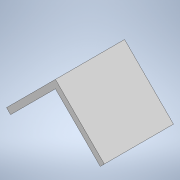
# Autodesk Inventor part: Tablero
Saved by Autodesk Inventor 2022 (Build 260153000, 153)
## iProperties
Created: 2022-08-25
Part Number: Tablero
Material: Generic
Document SubType Name: Modeling
Designer: Sebastian
Density: 1 g/cm^3
Appearance: Default
Author: Sebastian
Autodesk Inventor part; units mm, degrees
ref_plane "YZ Plane" through (0, 0, 0) normal (1, 0, 0) x (0, 1, 0)
ref_plane "XZ Plane" through (0, 0, 0) normal (0, 1, 0) x (-1, 0, 0)
ref_plane "XY Plane" through (0, 0, 0) normal (0, 0, 1) x (1, 0, 0)
sketch "Sketch1" plane through (0, 0, 0) normal (0, 0, 1) x (1, 0, 0)
  line L0 (0, 0) -> (-17.6777, 17.6777)
  line L1 (-17.6777, 17.6777) -> (194.4544, 229.8097)
  line L2 (-17.6777, 17.6777) -> (282.3223, 17.6777) construction
  line L3 (194.4544, 229.8097) -> (406.5864, 17.6777)
  line L4 (406.5864, 17.6777) -> (388.9087, 0)
  line L5 (388.9087, 0) -> (194.4544, 194.4544)
  line L6 (194.4544, 194.4544) -> (0, 0)
  dimension "d2" = 300
  dimension "d3" = 45
  dimension "d4" = 300
  dimension "d5" = 25
  constraints: 14 end point, 4 perpendicular, 1 equal length, 1 horizontal
  measures "d2" distance of L0.end L1.end
  measures "d3" angle of L2 L1
  measures "d4" distance of L1.end L3.end
  measures "d5" distance of L3.end L4.end
extrude "Extrusion1" add sketch "Sketch1" along normal blind 300
sketch "Sketch3" plane through (-17.6777, 17.6777, 0) normal (-0.7071, 0.7071, 0) x (-0.7071, -0.7071, 0)
  line L0 (-300, 0) -> (0, 0) projected
  line L1 (-180, 0) -> (-180, 300)
  line L2 (-300, 300) -> (0, 300) projected
  line L3 (-150, 0) -> (-180, 0)
  line L4 (-180, 0) -> (-180, 300)
  spline S0 degree 2 poles (-215.7606, 120.2254) (-207.5352, 120.2254) (-195.8732, 115.9437) (-188.4366, 107.8873) (-185, 96.3944) (-185, 88.4507) knots 0 0 0 1 2 3 4 4 4
  line L5 (-185, 88.4507) -> (-185, 74.1972)
  spline S1 degree 2 poles (-185, 74.1972) (-185, 72.6761) (-186.8028, 70.5915) (-188.831, 70.5915) knots 0 0 0 1 2 2 2
  line L6 (-188.831, 70.5915) -> (-240.8873, 70.5915)
  spline S2 degree 2 poles (-240.8873, 70.5915) (-242.9155, 70.5915) (-244.7183, 72.6761) (-244.7183, 74.1972) knots 0 0 0 1 2 2 2
  line L7 (-244.7183, 74.1972) -> (-244.7183, 89.5211)
  spline S3 degree 2 poles (-244.7183, 89.5211) (-244.7183, 97.5211) (-241, 108.6197) (-233.6197, 116.2817) (-222.8592, 120.2254) (-215.7606, 120.2254) knots 0 0 0 1 2 3 4 4 4
  spline S4 degree 2 poles (-215.3099, 107.662) (-219.5352, 107.662) (-226.8592, 105.6901) (-232.2113, 101.2958) (-235.1972, 94.4225) (-235.1972, 88.8451) knots 0 0 0 1 2 3 4 4 4
  line L8 (-235.1972, 88.8451) -> (-235.1972, 82.7042)
  line L9 (-235.1972, 82.7042) -> (-194.5775, 82.7042)
  line L10 (-194.5775, 82.7042) -> (-194.5775, 89.0141)
  spline S5 degree 2 poles (-194.5775, 89.0141) (-194.5775, 94.0282) (-197.169, 100.8451) (-202.3521, 105.4084) (-210.1268, 107.662) (-215.3099, 107.662) knots 0 0 0 1 2 3 4 4 4
  spline S6 degree 2 poles (-202.9155, 186.9296) (-198.1831, 186.9296) (-191.0845, 183.4366) (-186.3521, 177.4084) (-183.9296, 169.4084) (-183.9296, 164.8451) knots 0 0 0 1 2 3 4 4 4
  spline S7 degree 2 poles (-183.9296, 164.8451) (-183.9296, 161.7465) (-184.9437, 156.4507) (-186.4085, 152.3944) (-187.9859, 149.6338) (-189.169, 148.4507) (-191.4225, 147.9437) (-193.5634, 147.9437) knots 0 0 0 1 2 3 4 5 6 6 6
  spline S8 degree 2 poles (-193.5634, 147.9437) (-194.9718, 147.9437) (-196.9437, 148.1127) (-198.1268, 148.5634) (-198.6338, 149.2394) (-198.6338, 149.6901) knots 0 0 0 1 2 3 4 4 4
  spline S9 degree 2 poles (-198.6338, 149.6901) (-198.6338, 150.3662) (-197.1127, 152.6761) (-195.2535, 156.3944) (-193.7324, 161.5211) (-193.7324, 164.8451) knots 0 0 0 1 2 3 4 4 4
  spline S10 degree 2 poles (-193.7324, 164.8451) (-193.7324, 167.0986) (-194.8028, 170.5915) (-196.7183, 173.0141) (-199.5915, 174.3099) (-201.338, 174.3099) knots 0 0 0 1 2 3 4 4 4
  spline S11 degree 2 poles (-201.338, 174.3099) (-203.3662, 174.3099) (-206.2958, 172.1127) (-208.5493, 168.5634) (-210.5211, 164.0563) (-212.7183, 159.2113) (-215.5352, 154.7042) (-219.4789, 151.1549) (-224.831, 148.9577) (-228.5493, 148.9577) knots 0 0 0 1 2 3 4 5 6 7 8 8 8
  spline S12 degree 2 poles (-228.5493, 148.9577) (-232.8873, 148.9577) (-239.3662, 152.169) (-243.6479, 157.5211) (-245.7887, 164.9014) (-245.7887, 169.0141) knots 0 0 0 1 2 3 4 4 4
  spline S13 degree 2 poles (-245.7887, 169.0141) (-245.7887, 171.0986) (-245.169, 175.3803) (-244.0423, 179.0423) (-242.6338, 181.9155) (-241.7324, 182.8732) (-241.1127, 183.1549) (-240.0423, 183.3803) (-238.4085, 183.493) (-237.2254, 183.493) knots 0 0 0 1 2 3 4 5 6 7 8 8 8
  spline S14 degree 2 poles (-237.2254, 183.493) (-235.8732, 183.493) (-234.0141, 183.3803) (-232.831, 183.0423) (-232.2676, 182.4225) (-232.2676, 181.9155) knots 0 0 0 1 2 3 4 4 4
  spline S15 degree 2 poles (-232.2676, 181.9155) (-232.2676, 181.4084) (-233.5634, 179.2113) (-235.0845, 175.9437) (-236.3239, 171.7183) (-236.3239, 169.1831) knots 0 0 0 1 2 3 4 4 4
  spline S16 degree 2 poles (-236.3239, 169.1831) (-236.3239, 167.2113) (-235.3662, 164.2253) (-233.6197, 162.2535) (-231.2535, 161.2958) (-229.9014, 161.2958) knots 0 0 0 1 2 3 4 4 4
  spline S17 degree 2 poles (-229.9014, 161.2958) (-227.9296, 161.2958) (-225, 163.4366) (-222.7465, 167.0986) (-220.7746, 171.7183) (-218.5775, 176.507) (-215.7606, 181.1268) (-211.8169, 184.7324) (-206.5211, 186.9296) (-202.9155, 186.9296) knots 0 0 0 1 2 3 4 5 6 7 8 8 8
  spline S18 degree 2 poles (-201.6197, 235.8873) (-197.5634, 235.8873) (-191.0845, 234.3662) (-186.5211, 230.7042) (-184.0986, 224.7887) (-184.0986, 220.4507) knots 0 0 0 1 2 3 4 4 4
  spline S19 degree 2 poles (-184.0986, 220.4507) (-184.0986, 219.0986) (-184.493, 216.3944) (-185.169, 214.0845) (-185.9014, 212.4507) (-186.5211, 211.8873) (-187.1408, 211.5493) (-188.2113, 211.2676) (-189.7887, 211.1549) (-190.9718, 211.1549) knots 0 0 0 1 2 3 4 5 6 7 8 8 8
  spline S20 degree 2 poles (-190.9718, 211.1549) (-192.5493, 211.1549) (-194.7465, 211.2676) (-195.9859, 211.6056) (-196.493, 212.2253) (-196.493, 212.6761) knots 0 0 0 1 2 3 4 4 4
  spline S21 degree 2 poles (-196.493, 212.6761) (-196.493, 213.0704) (-195.8732, 214.1972) (-195.2535, 215.6056) (-194.6338, 217.4648) (-194.6338, 218.7042) knots 0 0 0 1 2 3 4 4 4
  spline S22 degree 2 poles (-194.6338, 218.7042) (-194.6338, 219.9437) (-195.3099, 221.8028) (-197.0563, 223.0986) (-199.8732, 223.7183) (-202.1268, 223.7183) knots 0 0 0 1 2 3 4 4 4
  line L11 (-202.1268, 223.7183) -> (-243.1408, 223.7183)
  spline S23 degree 2 poles (-243.1408, 223.7183) (-243.5915, 223.7183) (-244.3239, 224.338) (-244.7746, 225.6338) (-245, 228.0563) (-245, 229.8028) knots 0 0 0 1 2 3 4 4 4
  spline S24 degree 2 poles (-245, 229.8028) (-245, 231.5493) (-244.7746, 233.8592) (-244.3239, 235.2676) (-243.5915, 235.8873) (-243.1408, 235.8873) knots 0 0 0 1 2 3 4 4 4
  line L12 (-243.1408, 235.8873) -> (-201.6197, 235.8873)
  line L13 (-137.3875, 146.4329) -> (-137.3875, 162.5915)
  line L14 (-137.3875, 162.5915) -> (-130.2534, 162.5915)
  spline S25 degree 2 poles (-130.2534, 162.5915) (-129.8875, 177.3476) (-111.229, 195.6402) (-96.29, 195.6402) knots 0 0 0 1 2 2 2
  spline S26 degree 2 poles (-96.29, 195.6402) (-82.5095, 195.6402) (-62.6314, 178.2012) (-61.7778, 162.5915) knots 0 0 0 1 2 2 2
  line L15 (-61.7778, 162.5915) -> (-52.1436, 162.5915)
  line L16 (-52.1436, 162.5915) -> (-52.1436, 146.4329)
  line L17 (-52.1436, 146.4329) -> (-61.7778, 146.4329)
  spline S27 degree 2 poles (-61.7778, 146.4329) (-62.6314, 130.7622) (-82.5705, 113.3232) (-96.29, 113.3232) knots 0 0 0 1 2 2 2
  spline S28 degree 2 poles (-96.29, 113.3232) (-105.8022, 113.3232) (-120.5583, 120.8842) (-130.0095, 135.8842) (-130.2534, 146.4329) knots 0 0 0 1 2 3 3 3
  line L18 (-130.2534, 146.4329) -> (-137.3875, 146.4329)
  spline S29 degree 2 poles (-116.5339, 146.4329) (-115.7412, 138.9329) (-105.1924, 129.9695) (-96.29, 129.9695) knots 0 0 0 1 2 2 2
  spline S30 degree 2 poles (-96.29, 129.9695) (-87.9973, 129.9695) (-76.7778, 138.5671) (-76.0461, 146.4329) knots 0 0 0 1 2 2 2
  line L19 (-76.0461, 146.4329) -> (-116.5339, 146.4329)
  spline S31 degree 2 poles (-76.0461, 162.5915) (-76.8388, 170.0305) (-87.3266, 178.9939) (-96.29, 178.9939) knots 0 0 0 1 2 2 2
  spline S32 degree 2 poles (-96.29, 178.9939) (-104.5827, 178.9939) (-115.8632, 170.4573) (-116.5339, 162.5915) knots 0 0 0 1 2 2 2
  line L20 (-116.5339, 162.5915) -> (-76.0461, 162.5915)
  dimension "d8" = 30
  constraints: 6 end point, 2 point on line, 1 perpendicular, 1 vertical
  measures "d8" distance of L3.start L3.end
extrude "Extrusion2" cut sketch "Sketch3" against normal blind 5
body "Solid1"
